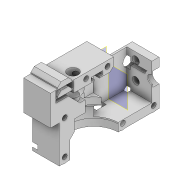
# Autodesk Inventor part: 10_SOOCT_Base_v3
Saved by Autodesk Inventor 2022 (Build 260153000, 153)
## iProperties
Created: 2023-01-02
Part Number: 10_SOOCT_Base_v3
Material: Generisch
Document SubType Name: Modeling
Designer: diederichbenedict
Density: 1 g/cm^3
Appearance: Vorgabe
Author: diederichbenedict
Autodesk Inventor part; units mm, degrees
ref_plane "YZ Plane" through (0, 0, 0) normal (1, 0, 0) x (0, 1, 0)
ref_plane "XZ Plane" through (0, 0, 0) normal (0, 1, 0) x (-1, 0, 0)
ref_plane "XY Plane" through (0, 0, 0) normal (0, 0, 1) x (1, 0, 0)
ref_plane "Arbeitsebene1" through (-39.7131, -1.3218, -40.6417) normal (-1, 0, 0) x (0, 0, -1)
sketch "Skizze1" plane through (-39.7131, -1.3218, -40.6417) normal (-1, 0, 0) x (0, 0, -1)
  line L0 (-10.1, 42.0592) -> (-10.1, 20.2092)
  line L1 (-10.1, 19.2092) -> (-10.1, 18.0592)
  line L2 (-37.1, 42.0592) -> (-37.1, 20.2092)
  line L3 (-37.1, 19.2092) -> (-37.1, 18.0592)
  line L4 (4, 5) -> (1, 5)
  line L5 (-37.1, 27.2) -> (-43.1, 27.2)
  line L6 (-43.1, 27.2) -> (-43.1, 3.2)
  line L7 (-43.1, 3.2) -> (-37.1, 3.2)
  line L8 (-37.1, 3.2) -> (-37.1, 27.2)
  line L9 (-7.8, 3.2) -> (0, 3.2)
  line L10 (-37.1, 3.2) -> (12.9, 3.2)
  line L11 (12.9, 3.2) -> (12.9, 27.2)
  line L12 (12.9, 27.2) -> (-37.1, 27.2)
  line L13 (-37.1, 27.2) -> (-37.1, 3.2)
  point P0 (-40.6417, -1.3218)
  point P1 (-37.1, 24.2092)
  point P2 (-7.8, 3.2)
  dimension "d0" = 0
  dimension "d2" = 6
  dimension "d3" = 50
  dimension "d21" = 24
  constraints: 28 end point, 4 horizontal, 4 parallel, 4 vertical, 2 perpendicular, 1 point on line, 12 other
  measures "d0" distance between parallel lines of L7 L9
  measures "d2" distance between parallel lines of L8 L6
  measures "d3" distance of L5.start L11.end
  measures "d21" distance between parallel lines of L12 L7
extrude "Extrusion1" add sketch "Skizze1" against normal up to surface (17 mm away)
sketch "Skizze2" plane through (-22.7131, -28.5218, 2.4583) normal (1, 0, 0) x (0, 0, -1)
  line L0 (33, 5) -> (33, 6.15)
  line L1 (33, -17.85) -> (33, 4)
  line L2 (0, 24) -> (56, 24)
  line L3 (8.5007, 24) -> (8.5007, 11.4732)
  line L4 (8.5007, 11.4732) -> (5.9, 8.8725)
  line L5 (5.9, 8.8725) -> (5.9, 7.6275)
  arc A0 (5.9, 6.8275) -> (5.9, 7.6275) centre (5.9, 7.2275) ccw
  line L6 (5.9, 6.8275) -> (5.9, -14.594)
  line L7 (56.2565, 0) -> (0.3327, 0)
  line L8 (15.7023, 20.4) -> (24.9625, 20.4029)
  line L9 (19.4614, 24) -> (19.4689, 0)
  line L10 (33, 7.9908) -> (6, 7.9908) projected
  line L11 (33, 6.9908) -> (6, 6.9908) projected
  line L12 (56, 24) -> (0, 24) projected
  line L13 (6, 7.9908) -> (6, 9.1408)
  line L14 (56, 0) -> (56, 24) projected
  line L15 (56, 24) -> (0, 24) projected
  line L16 (0, 24) -> (0, 0) projected
  line L17 (0, 0) -> (56, 0) projected
  line L18 (5.9662, 8.7775) -> (13.9636, 16.7801)
  line L19 (5.9, 7.6275) -> (5.9, 6.8275)
  point P0 (2.4583, 28.5218)
  point P1 (5.9, 0)
  point P2 (7.3142, 24)
  dimension "d10" = 5.5
  dimension "d37" = 0
  dimension "d38" = 0.1
  dimension "d39" = 0
  dimension "d40" = 0.8
  constraints: 26 end point, 6 point on line, 2 collinear, 2 point on circle, 1 centre point, 1 coincident, 1 parallel, 1 vertical, 4 other
  measures "d10" distance from line of L8.end L9
  measures "d37" distance between parallel lines of L12 L2
  measures "d38" distance between parallel lines of L13 L5
  measures "d39" distance between parallel lines of L6 L5
  measures "d40" distance of L5.end L6.start
revolve "Umdrehung1" cut sketch "Skizze2" angle 360 about axis through (-22.7131, -4.5218, -17.0031) along (0, -1, -0.0003154) contours L2 L9 L10 L13 L4 L3 | L13 L10 L9 L11 A0 L5 L4 | L6 A0 L11 L9 L7 | L19 A0
sketch "Skizze3" plane through (-22.7131, -28.5218, -53.5417) normal (1, 0, 0) x (0, 0, -1)
  line L0 (-38.5, 18.2) -> (-38.5, 22.2) projected
  line L1 (-34.5, 18.2) -> (-38.5, 18.2) projected
  line L2 (-34.5, 22.2) -> (-34.5, 18.2) projected
  line L3 (-38.5, 22.2) -> (-34.5, 22.2) projected
  line L4 (-34, 22.7) -> (-34, 17.7)
  line L5 (-34, 17.7) -> (-39, 17.7)
  line L6 (-39, 17.7) -> (-39, 22.7)
  line L7 (-39, 22.7) -> (-34, 22.7)
  line L8 (-47.4993, 11.4732) -> (-47.4993, 24) projected
  line L9 (-25.578, 24) -> (-25.5701, 11.4801) projected
  line L10 (-47.4993, 22.7) -> (-25.574, 22.7)
  line L11 (-25.574, 22.7) -> (-25.574, 17.7)
  line L12 (-25.574, 17.7) -> (-47.4993, 17.7)
  line L13 (-47.4993, 17.7) -> (-47.4993, 22.7)
  line L14 (-47.4993, 22.7) -> (-25.578, 22.7)
  line L15 (-25.578, 22.7) -> (-25.578, 24)
  line L16 (-25.578, 24) -> (-47.4993, 24)
  line L17 (-47.4993, 24) -> (-47.4993, 22.7)
  point P0 (-53.5417, 28.5218)
  point P1 (-47.4993, 17.7)
  point P2 (-34, 14.7092)
  point P3 (-25.5771, 22.7)
  point P4 (-34, 19.7092)
  point P5 (-34, 19.7092)
  point P6 (-34, 22.7)
  point P7 (-34, 17.7)
  point P8 (-47.4993, 24)
  point P9 (-25.578, 22.7)
  dimension "d12" = 0.5
  constraints: 24 end point, 4 parallel, 4 point on line, 2 horizontal, 2 perpendicular, 3 other
  measures "d12" distance between parallel lines of L3 L7
extrude "Extrusion2" add sketch "Skizze3" against normal through all contours L0 L3 L2 L1 | L10 L9 L12 L4 | L4 L5 L6 L7 | L7 L10 L8 L16 L9 | L6 L12 L8 L10 | L10 L11 L9
sketch "Skizze4" plane through (-22.7131, -28.5218, -53.5417) normal (1, 0, 0) x (0, 0, -1)
  line L0 (-38.5, 18.2) -> (-38.5, 22.2) projected
  line L1 (-34.5, 18.2) -> (-38.5, 18.2) projected
  line L2 (-34.5, 22.2) -> (-34.5, 18.2) projected
  line L3 (-38.5, 22.2) -> (-34.5, 22.2) projected
  line L4 (-34.45, 22.25) -> (-34.45, 18.15)
  line L5 (-34.45, 18.15) -> (-38.55, 18.15)
  line L6 (-38.55, 18.15) -> (-38.55, 22.25)
  line L7 (-38.55, 22.25) -> (-34.45, 22.25)
  line L8 (-56, 0) -> (-50.1, 0) projected
  line L9 (0, 0) -> (0, 24) projected
  line L10 (0, 24) -> (-25.578, 24) projected
  line L11 (-56, 24) -> (-56, 0) projected
  line L12 (-38.2, 22.25) -> (-34.8, 22.25)
  line L13 (-34.8, 22.25) -> (-34.8, 22.7)
  line L14 (-34.8, 22.7) -> (-38.2, 22.7)
  line L15 (-38.2, 22.7) -> (-38.2, 22.25)
  line L16 (-34.5, 18.2) -> (-34.5, 22.2)
  line L17 (-38.25, 18.15) -> (-34.75, 18.15)
  line L18 (-34.75, 18.15) -> (-34.75, 17.7)
  line L19 (-34.75, 17.7) -> (-38.25, 17.7)
  line L20 (-38.25, 17.7) -> (-38.25, 18.15)
  line L21 (-25.578, 24) -> (-25.5771, 22.7) projected
  line L22 (-25.5701, 11.4801) -> (-22.9677, 8.8811) projected
  line L23 (-47.4993, 11.4732) -> (-47.4993, 17.7) projected
  line L24 (-50.1, 8.8725) -> (-47.4993, 11.4732) projected
  line L25 (-47.4993, 17.7) -> (-25.574, 17.7) projected
  line L26 (-25.574, 17.7) -> (-25.5701, 11.4801) projected
  line L27 (-25.5771, 22.7) -> (-25.578, 22.7) projected
  line L28 (-22.9621, 0.0086) -> (-36.5311, 0) projected
  line L29 (-36.5311, 0) -> (0, 0) projected
  line L30 (-25.578, 22.7) -> (-25.578, 24) projected
  line L31 (-25.578, 24) -> (-56, 24) projected
  line L32 (-38.2, 22.7) -> (-34.8, 22.7)
  line L33 (-34.8, 22.7) -> (-34.8, 24)
  line L34 (-34.8, 24) -> (-38.2, 24)
  line L35 (-38.2, 24) -> (-38.2, 22.7)
  line L36 (-34.45, 21.95) -> (-21.9312, 21.95)
  line L37 (-21.9312, 21.95) -> (-21.9312, 18.5)
  line L38 (-21.9312, 18.5) -> (-34.45, 18.5)
  line L39 (-34.45, 18.5) -> (-34.45, 21.95)
  line L40 (-50.1, 0) -> (-50.1, 8.8725) projected
  line L41 (-22.9677, 8.8811) -> (-22.9621, 0.0086) projected
  point P0 (-53.5417, 28.5218)
  point P1 (-43.6858, 14.7092)
  point P2 (-19.3142, 14.7092)
  point P3 (-47.4993, 22.7)
  point P4 (-34.75, 18.15)
  point P5 (-34.8059, 22.7)
  point P6 (-34.45, 18.5)
  dimension "d15" = 0.05
  dimension "d58" = 0.3
  dimension "d59" = 0.3
  dimension "d60" = 0.3
  dimension "d61" = 0.3
  dimension "d64" = 0.3
  dimension "d65" = 0.3
  constraints: 42 end point, 8 parallel, 5 point on line, 4 horizontal, 4 perpendicular, 3 other
  measures "d15" distance between parallel lines of L3 L7
  measures "d58" distance between parallel lines of L0 L15
  measures "d59" distance between parallel lines of L2 L33
  measures "d60" distance between parallel lines of L4 L18
  measures "d61" distance between parallel lines of L20 L6
  measures "d64" distance between parallel lines of L7 L36
  measures "d65" distance between parallel lines of L38 L1
extrude "Extrusion3" cut sketch "Skizze4" against normal blind 2 contours L0 L3 L2 L1 | L4 L5 L6 L7 | L36 L37 L38 L4 | L7 L15 L14 L13 | L14 L35 L31 L33 | L18 L19 L20 L5
sketch "Skizze5" plane through (-39.7131, -28.5218, -53.5417) normal (0, 0, -1) x (-1, 0, 0)
  arc A0 (-8, 26.2) -> (-9, 27.2) centre (-9, 26.2) ccw projected
  line L0 (-25, 27.2) -> (-9, 27.2) projected
  arc A1 (-25, 27.2) -> (-26, 26.2) centre (-25, 26.2) ccw projected
  line L1 (-26, 10.2) -> (-26, 26.2) projected
  arc A2 (-26, 10.2) -> (-25, 9.2) centre (-25, 10.2) ccw projected
  line L2 (-9, 9.2) -> (-25, 9.2) projected
  arc A3 (-9, 9.2) -> (-8, 10.2) centre (-9, 10.2) ccw projected
  line L3 (-8, 26.2) -> (-8, 10.2) projected
  circle A4 centre (-17, 18.2) radius 5.8 projected
  arc A5 (-9, 8.2) -> (-7, 10.2) centre (-9, 10.2) ccw
  line L4 (-9, 8.2) -> (-25, 8.2)
  arc A6 (-27, 10.2) -> (-25, 8.2) centre (-25, 10.2) ccw
  line L5 (-27, 10.2) -> (-27, 26.2)
  arc A7 (-25, 28.2) -> (-27, 26.2) centre (-25, 26.2) ccw
  line L6 (-25, 28.2) -> (-9, 28.2)
  arc A8 (-7, 26.2) -> (-9, 28.2) centre (-9, 26.2) ccw
  line L7 (-7, 26.2) -> (-7, 10.2)
  line L8 (-31, 32.2) -> (-3, 32.2)
  line L9 (-3, 32.2) -> (-3, 4.2)
  line L10 (-3, 4.2) -> (-31, 4.2)
  line L11 (-31, 4.2) -> (-31, 32.2)
  line L12 (-31, 32.2) -> (-3, 4.2) construction
  line L13 (-3, 32.2) -> (-31, 4.2) construction
  point P0 (-39.7131, 28.5218)
  dimension "d18" = 1
  dimension "d27" = 28
  dimension "d28" = 28
  constraints: 20 end point, 8 point on circle, 4 centre point, 2 midpoint, 2 parallel, 1 horizontal, 1 perpendicular, 7 other
  measures "d18" distance between parallel lines of L3 L7
  measures "d27" distance of L9.end L10.end
  measures "d28" distance of L8.end L9.end
extrude "Extrusion4" cut sketch "Skizze5" against normal blind 20 contours L3 A3 L2 A2 L1 A1 L0 A0 | A4 | L4 A6 L5 A7 L6 A8 L7 A5
sketch "Skizze6" plane through (-39.7131, -28.5218, -53.5417) normal (0, 0, -1) x (-1, 0, 0)
  line L0 (-9, 8.2) -> (-17, 8.2) projected
  line L1 (-17, 0) -> (-17, 8.2) projected
  line L2 (0, 0) -> (-17, 0) projected
  line L3 (0, 24) -> (0, 0) projected
  line L4 (0, 24) -> (-7, 24) projected
  line L5 (-7, 24) -> (-7, 10.2) projected
  arc A0 (-9, 8.2) -> (-7, 10.2) centre (-9, 10.2) ccw projected
  line L6 (-17, 8.2) -> (-17, 11.4801) projected
  line L7 (-17, 8.2) -> (-7, 8.2)
  line L8 (-7, 8.2) -> (-7, 24)
  line L9 (-7, 24) -> (-17, 24)
  line L10 (-17, 24) -> (-17, 8.2)
  circle A1 centre (-17, 18.2) radius 4 projected
  circle A2 centre (-17, 15.0113) radius 4
  point P0 (-39.7131, 28.5218)
  point P1 (-17, 22.2)
  point P2 (-17, 14.2)
  point P3 (-17, 19.0113)
  point P4 (-17, 11.0113)
  constraints: 8 end point, 2 parallel, 1 centre point, 1 horizontal, 1 perpendicular, 2 other
ref_plane "Arbeitsebene2" through (-26.7131, -14.3218, -41.6417) normal (0, 0, 1) x (1, 0, 0)
ref_plane "Arbeitsebene3" through (-26.7131, -14.3218, -44.6417) normal (0, 0, -1) x (0, 1, 0)
extrude "Extrusion5" add sketch "Skizze6" against normal blind 8 contours L0 L6 A2 A1 L10 L9 L5 A0 | A1 A2 L10 picked at (-16.3965, 20.005)
sketch "Skizze7" plane through (-32.7131, -4.5218, -45.5417) normal (0, 0, 1) x (1, 0, 0)
  circle A0 centre (10, -5.8) radius 4
  line L0 (10, 0) -> (10, -24) projected
  line L1 (10, -9.8) -> (10, -1.8)
  circle A1 centre (10, -5.8) radius 3
  circle A2 centre (10, -8.9887) radius 4 projected
  point P0 (32.7131, 4.5218)
  point P1 (10, -8.8)
  point P2 (10, -2.8)
  dimension "d24" = 1
  constraints: 2 centre point, 2 end point, 1 point on circle
  measures "d24" radial gap between concentric circles of A0 A1
extrude "Extrusion6" add sketch "Skizze7" against normal blind 0.5 contours L0 A1 A2 A0 | A2 A1 L0 A0 picked at (9.6732, -2.174) picked at (9.6932, -9.4309)
ref_plane "Arbeitsebene4" through (-39.7131, -28.5218, -35.5417) normal (0, 0, -1) x (-1, 0, 0)
sketch "Skizze8" plane through (-39.7131, -28.5218, -35.5417) normal (0, 0, -1) x (-1, 0, 0)
  circle A0 centre (-17, 18.2) radius 4 projected
  line L0 (-3, 3.7) -> (-31, 3.7)
  line L1 (-31, 3.7) -> (-31, 32.7)
  line L2 (-31, 32.7) -> (-3, 32.7)
  line L3 (-3, 32.7) -> (-3, 3.7)
  line L4 (-17, 22.2) -> (-17, 18.2) projected
  line L5 (-3, 3.7) -> (-31, 32.7) construction
  line L6 (-31, 3.7) -> (-3, 32.7) construction
  point P0 (-39.7131, 28.5218)
  dimension "d30" = 28
  dimension "d31" = 29
  constraints: 12 end point, 2 midpoint, 2 parallel, 1 horizontal, 1 perpendicular, 1 vertical alignment
  measures "d30" distance of L1.end L2.end
  measures "d31" distance of L0.end L1.end
extrude "Extrusion7" cut sketch "Skizze8" along normal blind 14 and the other way blind 9 contours A0 | L0 L1 L2 L3
sketch "Skizze9" plane through (-39.7131, -28.5218, -53.5417) normal (0, 0, -1) x (-1, 0, 0)
  line L0 (-17, 11.0113) -> (-17, 0) projected
  line L1 (0, 0) -> (-17, 0) projected
  line L2 (0, 24) -> (0, 0) projected
  line L3 (0, 24) -> (-17, 24) projected
  line L4 (-17, 24) -> (-17, 19.0113) projected
  arc A0 (-17, 11.0113) -> (-17, 19.0113) centre (-17, 15.0113) ccw projected
  line L5 (-26, 10.0113) -> (-8, 10.0113)
  line L6 (-8, 10.0113) -> (-8, 20.0113)
  line L7 (-8, 20.0113) -> (-26, 20.0113)
  line L8 (-26, 20.0113) -> (-26, 10.0113)
  line L9 (-26, 10.0113) -> (-8, 20.0113) construction
  line L10 (-8, 10.0113) -> (-26, 20.0113) construction
  circle A1 centre (-8, 20.0113) radius 2
  circle A2 centre (-8, 10.0113) radius 2
  point P0 (-39.7131, 28.5218)
  dimension "d99" = 18
  dimension "d100" = 10
  dimension "d101" = 4
  dimension "d102" = 4
  constraints: 12 end point, 2 centre point, 2 coincident, 2 midpoint, 2 parallel, 1 horizontal, 1 perpendicular
  measures "d99" distance of L7.end L6.end
  measures "d100" distance of L6.end L5.end
  measures "d101" diameter of A1
  measures "d102" diameter of A2
extrude "Extrusion8" cut sketch "Skizze9" against normal blind 14 contours A2 L6 L5 | L5 L6 A2 | A1 L6 L7 | L7 L6 A1
sketch "Skizze10" plane through (-39.7131, -28.5218, -53.5417) normal (0, -1, 0) x (1, 0, 0)
  line L0 (8.5019, 6.0924) -> (3.4981, 6.0924) projected
  line L1 (17, 56) -> (17, 50.1) projected
  line L2 (0, 56) -> (17, 56) projected
  line L3 (0, 0) -> (0, 56) projected
  line L4 (0, 0) -> (17, 0) projected
  line L5 (17, 36.5311) -> (17, 0) projected
  line L6 (17, 50.1) -> (17, 36.5311) projected
  ellipse E0 centre (17, 36.5311) end of major axis (30.5689, 36.5311) minor radius 13.5689 (17, 50.1) -> (17, 22.9621) ccw projected
  point P0 (39.7131, 53.5417)
  constraints: 1 other
extrude "Extrusion9" cut sketch "Skizze10" against normal blind 3 contours L6 L5 E0
sketch "Skizze11" plane through (-39.7131, -28.5218, -53.5417) normal (0, -1, 0) x (1, 0, 0)
  circle A0 centre (17, 36.5) radius 13.5 projected
  ellipse E0 centre (17, 36.5311) end of major axis (30.5689, 36.5311) minor radius 13.5689 (17, 50.1) -> (17, 22.9621) ccw projected
  line L0 (17, 56) -> (17, 50.1) projected
  line L1 (0, 56) -> (17, 56) projected
  line L2 (0, 0) -> (0, 56) projected
  line L3 (0, 0) -> (17, 0) projected
  line L4 (17, 22.9621) -> (17, 0) projected
  point P0 (39.7131, 53.5417)
  constraints: 1 other
extrude "Extrusion10" add sketch "Skizze11" along normal blind 3 contours E0 L4 L3 L2 L1 L0
sketch "Skizze12" plane through (-39.7131, -1.3218, -40.6417) normal (-1, 0, 0) x (0, 0, 1)
  circle A0 centre (40.1, -25.2) radius 1.29
  circle A1 centre (40.1, -6.2) radius 1.4
  circle A2 centre (-9.9, -25.2) radius 1.4
  circle A3 centre (7.4249, -25.2) radius 1.4
  circle A4 centre (-9.9, -10.2) radius 1.4
  line L0 (43.1, -30.2) -> (-12.9, -30.2) projected
  line L1 (43.1, -30.2) -> (43.1, -3.2) projected
  line L2 (-12.9, -3.2) -> (-12.9, -30.2) projected
  line L3 (43.1, -3.2) -> (-12.9, -3.2) projected
  point P0 (40.6417, 1.3218)
  dimension "d46" = 2.58
  dimension "d47" = 2.8
  dimension "d48" = 2.8
  dimension "d49" = 2.8
  dimension "d50" = 2.8
  dimension "d90" = 3
  dimension "d91" = 3
  dimension "d92" = 3
  dimension "d93" = 5
  dimension "d94" = 5
  dimension "d95" = 5
  dimension "d96" = 3
  dimension "d97" = 7
  dimension "d98" = 3
  constraints: 5 centre point
  measures "d46" diameter of A0
  measures "d47" diameter of A1
  measures "d48" diameter of A2
  measures "d49" diameter of A3
  measures "d50" diameter of A4
  measures "d90" distance from line of A0.centre L1
  measures "d91" distance from line of A1.centre L1
  measures "d92" distance from line of L3 A1.centre
  measures "d93" distance from line of L0 A0.centre
  measures "d94" distance from line of L0 A3.centre
  measures "d95" distance from line of L0 A2.centre
  measures "d96" distance from line of A4.centre L2
  measures "d97" distance from line of A4.centre L3
  measures "d98" distance from line of L2 A2.centre
hole "Bohrung1" at (-39.7131, -26.5218, -0.5417) at (-39.7131, -7.5218, -0.5417) at (-39.7131, -26.5218, -33.2168) at (-39.7131, -26.5218, -50.5417) at (-39.7131, -11.5218, -50.5417) direction (1, 0, 0) diameter 2.8 end through all counterbore diameter 6.5 counterbore depth 5
sketch "Skizze13" plane through (-39.7131, -1.3218, -40.6417) normal (-1, 0, 0) x (0, 0, 1)
  line L0 (37.2, -30.2) -> (43.1, -30.2) projected
  line L1 (43.1, -30.2) -> (-14.489, -30.2)
  line L2 (-14.489, -30.2) -> (-14.489, -1.9274)
  line L3 (-14.489, -1.9274) -> (43.1, -1.9274)
  line L4 (43.1, -1.9274) -> (43.1, -30.2)
  point P0 (40.6417, 1.3218)
  point P1 (37.2, -30.2)
  constraints: 8 end point, 2 parallel, 1 horizontal, 1 perpendicular
extrude "Extrusion11" cut sketch "Skizze13" against normal blind 2
sketch "Skizze14" plane through (-39.7131, -28.5218, -49.5417) normal (0, 0, 1) x (1, 0, 0)
  arc A0 (17, 19.0113) -> (17, 11.0113) centre (17, 15.0113) ccw projected
  circle A1 centre (17, 15.0113) radius 2.5
  line L0 (17, 11.0113) -> (17, 3.7) projected
  line L1 (17, 11.0113) -> (17, 19.0113)
  point P0 (39.7131, 28.5218)
  point P1 (17, 9.4504)
  point P2 (17, 12.5113)
  point P3 (17, 17.5113)
  dimension "d68" = 5
  constraints: 2 end point, 1 centre point, 1 coincident, 1 collinear
  measures "d68" diameter of A1
extrude "Extrusion12" add sketch "Skizze14" against normal blind 0.5 contours L1 A1 A0
sketch "Skizze15" plane through (-37.7131, -1.3218, -40.6417) normal (-1, 0, 0) x (0, 0, 1)
  circle A0 centre (7.4249, -25.2) radius 3.25 projected
  arc A1 (38.85, -3.2) -> (43.1, -7.45) centre (40.1, -6.2) ccw projected
  line L0 (43.1, -3.2) -> (43.1, -4.95) projected
  line L1 (-12.9, -8.95) -> (-12.9, -3.2) projected
  line L2 (-12.9, -30.2) -> (-12.9, -26.45) projected
  line L3 (43.1, -26.45) -> (43.1, -30.2) projected
  line L4 (43.1, -3.2) -> (43.1, -30.2) projected
  line L5 (-12.9, -30.2) -> (43.1, -30.2)
  line L6 (43.1, -30.2) -> (43.1, -28.2)
  line L7 (43.1, -28.2) -> (-12.9, -28.2)
  line L8 (-12.9, -28.2) -> (-12.9, -30.2)
  arc A2 (43.1, -4.95) -> (41.35, -3.2) centre (40.1, -6.2) ccw projected
  arc A3 (-12.9, -11.45) -> (-12.9, -8.95) centre (-9.9, -10.2) ccw projected
  line L9 (41.35, -3.2) -> (43.1, -3.2) projected
  arc A4 (43.1, -23.95) -> (43.1, -26.45) centre (40.1, -25.2) ccw projected
  line L10 (43.1, -30.2) -> (-12.9, -30.2) projected
  line L11 (43.1, -7.45) -> (43.1, -23.95) projected
  line L12 (-12.9, -3.2) -> (38.85, -3.2) projected
  arc A5 (-12.9, -26.45) -> (-12.9, -23.95) centre (-9.9, -25.2) ccw projected
  line L13 (-12.9, -23.95) -> (-12.9, -11.45) projected
  point P0 (40.6417, 1.3218)
  point P1 (6.1749, -28.2)
  point P2 (8.6749, -28.2)
  point P3 (41.35, -30.2)
  point P4 (43.1, -28.45)
  point P5 (0.4177, -30.2)
  point P6 (2.9177, -30.2)
  point P7 (2.9177, -30.2)
  point P8 (-12.9, -28.45)
  point P9 (-11.15, -30.2)
  point P10 (-8.65, -28.2)
  point P11 (-11.15, -28.2)
  point P12 (41.35, -28.2)
  point P13 (38.85, -28.2)
  dimension "d71" = 2
  constraints: 8 end point, 2 parallel, 1 horizontal, 1 perpendicular, 1 point on line
  measures "d71" distance of L6.end L5.end
extrude "Extrusion13" cut sketch "Skizze15" against normal through all contours A0 L7 A4 L3 L5 L2 A5
sketch "Skizze16" plane through (-22.7131, -20.8943, -3.4417) normal (1, 0, 0) x (0, 0, -1)
  circle A0 centre (13.6, 12.5725) radius 4.6
  line L0 (50.1, 16.3725) -> (-5.9, 16.3725) projected
  line L1 (9.9503, 16.3725) -> (9.9503, 15.3725)
  line L2 (9.9503, 16.3725) -> (10.9503, 16.3725) construction
  line L3 (17.2497, 16.3725) -> (17.2497, 15.3725)
  line L4 (11.55, 14.6225) -> (15.65, 10.5225)
  line L5 (15.65, 10.5225) -> (15.65, 14.6225)
  line L6 (15.65, 14.6225) -> (11.55, 10.5225)
  point P0 (-3.4417, 20.8943)
  point P1 (16.1923, 16.3725)
  point P2 (11.0077, 16.3725)
  dimension "d74" = 9.2
  dimension "d80" = 90
  dimension "d81" = 1
  dimension "d82" = 1
  constraints: 12 end point, 3 midpoint, 2 perpendicular, 2 point on circle, 2 point on line, 2 vertical, 1 centre point, 1 horizontal
  measures "d74" diameter of A0
  measures "d80" angle of L1 L2
  measures "d81" distance of L1.end L1.start
  measures "d82" distance from line of L3.end L0
extrude "Extrusion14" cut sketch "Skizze16" against normal blind 13 contours A0 L0 | A0 L0 L3 | L1 L0 A0 | L0 A0 | L6 L5 L4
ref_plane "Arbeitsebene5" through (-32.7131, -12.3218, -21.0417) normal (1, 0, 0) x (0, 1, 0)
sketch "Skizze18" plane through (-22.7131, -20.8943, -3.4417) normal (1, 0, 0) x (0, 0, -1)
  line L0 (9.9503, 15.3725) -> (9.9503, 16.3725) projected
  line L1 (9.9503, 16.3725) -> (-5.9, 16.3725) projected
  line L2 (-5.9, 16.3725) -> (-5.9, -8.6275) projected
  line L3 (0, -4.6275) -> (0, -8.6275) projected
  line L4 (0, 1.245) -> (2.6007, 3.8457) projected
  line L5 (2.6007, 3.8457) -> (2.6007, 10.0725) projected
  line L6 (2.6007, 10.0725) -> (9.7387, 10.0725) projected
  arc A0 (9.9503, 15.3725) -> (9.7387, 10.0725) centre (13.6, 12.5725) ccw projected
  circle A1 centre (-2.9, -5.6275) radius 1.4 projected
  circle A2 centre (-2.9, 13.3725) radius 1.4 projected
  line L7 (18.5632, 7.5725) -> (8.5632, 7.5725)
  line L8 (8.5632, 7.5725) -> (8.5632, 17.5725)
  line L9 (8.5632, 17.5725) -> (18.5632, 17.5725)
  line L10 (18.5632, 17.5725) -> (18.5632, 7.5725)
  line L11 (18.5632, 7.5725) -> (8.5632, 17.5725) construction
  line L12 (8.5632, 7.5725) -> (18.5632, 17.5725) construction
  line L13 (50.1, 3.3838) -> (50.1, -8.6275) projected
  line L14 (46.1, -3.9275) -> (46.1, 4.8838) projected
  line L15 (46.1, -3.9275) -> (27.1355, -3.9275) projected
  line L16 (27.1355, -3.9275) -> (27.136, -4.6275) projected
  line L17 (27.136, -4.6275) -> (27.1379, -4.6275) projected
  line L18 (27.1379, -4.6275) -> (27.1379, -8.6275) projected
  circle A3 centre (29.7751, -5.6275) radius 1.4 projected
  circle A4 centre (47.1, -5.6275) radius 1.4 projected
  line L19 (50.1, 3.3838) -> (46.6, 3.3838) projected
  line L20 (46.6, 4.8838) -> (46.6, 3.3838) projected
  line L21 (46.1, 4.8838) -> (46.6, 4.8838) projected
  line L22 (48.35, -8.6275) -> (50.1, -8.6275) projected
  line L23 (27.1379, -8.6275) -> (28.5251, -8.6275) projected
  arc A5 (28.5251, -8.6275) -> (31.0251, -8.6275) centre (29.7751, -5.6275) ccw projected
  line L24 (31.0251, -8.6275) -> (45.85, -8.6275) projected
  arc A6 (45.85, -8.6275) -> (48.35, -8.6275) centre (47.1, -5.6275) ccw projected
  line L25 (-5.9, -8.6275) -> (-4.15, -8.6275) projected
  arc A7 (-4.15, -8.6275) -> (-1.65, -8.6275) centre (-2.9, -5.6275) ccw projected
  line L26 (-1.65, -8.6275) -> (0, -8.6275) projected
  line L27 (18.5632, 7.5725) -> (24.0476, 7.5725)
  line L28 (24.0476, 7.5725) -> (24.0476, 17.5725)
  line L29 (24.0476, 17.5725) -> (18.5632, 17.5725)
  line L30 (18.5632, 17.5725) -> (18.5632, 7.5725)
  line L31 (0, -4.6275) -> (0, 1.245) projected
  point P0 (-3.4417, 20.8943)
  point P1 (13.5632, 12.5725)
  point P2 (8.5632, 10.0725)
  point P3 (8.5632, 16.3725)
  dimension "d83" = 10
  dimension "d84" = 10
  constraints: 20 end point, 4 parallel, 2 horizontal, 2 midpoint, 2 perpendicular
  measures "d83" distance of L8.end L9.end
  measures "d84" distance of L7.end L8.end
extrude "Extrusion16" cut sketch "Skizze18" against normal up to surface (10 mm away) contours A0 L6 L8 L1 L0 | L0 L1 L8 L9 L10 L7 L6 A0 | L29 L28 L27 L10
sketch "Skizze19" plane through (-37.7131, -1.3218, -40.6417) normal (-1, 0, 0) x (0, 0, 1)
  circle A0 centre (23.6, -7) radius 1.5 projected
  circle A1 centre (23.6, -7) radius 1.6
  point P0 (40.6417, 1.3218)
  dimension "d87" = 3.2
  constraints: 1 centre point, 1 coincident
  measures "d87" diameter of A1
extrude "Extrusion17" cut sketch "Skizze19" against normal through all contours A0 | A1
sketch "Skizze20" plane through (-34.7131, -8.7718, 2.4583) normal (0, 0, 1) x (1, 0, 0)
  line L0 (2.55, -2.9214) -> (5.65, -2.9214) construction
  line L1 (5.65, -2.9214) -> (2.55, -2.9214) projected
  line L2 (2.2436, -4.55) -> (2.2441, -2.05) projected
  line L3 (2.2441, -2.05) -> (12, -2.05) projected
  line L4 (2.55, -2.9214) -> (2.55, 0.1786) construction
  line L5 (2.55, 0.1786) -> (5.65, 0.1786) projected
  line L6 (12, 4.25) -> (12, -20.75) projected
  line L7 (-3, 4.25) -> (12, 4.25) projected
  line L8 (-3, 4.25) -> (-3, 2.5) projected
  line L9 (-3, 2.5) -> (0, 2.5) projected
  line L10 (0, 2.5) -> (0, 0) projected
  line L11 (0, 0) -> (-3, 0) projected
  line L12 (-3, 0) -> (-3, -16.5) projected
  line L13 (-3, -16.5) -> (0, -16.5) projected
  line L14 (0, -16.5) -> (0, -19) projected
  line L15 (5.65, 0.1786) -> (5.65, -2.9214) projected
  circle A0 centre (4.1, -1.7586) radius 1.55
  circle A1 centre (4.1, -1.7586) radius 2
  line L16 (14.05, -1.65) -> (9.95, -1.65) projected
  line L17 (9.95, 2.55) -> (9.95, -1.65) projected
  line L18 (9.95, 2.55) -> (14.05, 2.55) projected
  line L19 (14.05, 2.55) -> (14.05, -1.65) projected
  line L20 (0, -19) -> (-3, -19) projected
  line L21 (-3, -19) -> (-3, -20.75) projected
  line L22 (-3, -20.75) -> (12, -20.75) projected
  point P0 (34.7131, 8.7718)
  point P1 (5.8244, -2.15)
  point P2 (2.8244, -2.15)
  dimension "d103" = 4
  constraints: 2 centre point, 2 end point, 1 coincident, 6 other
  measures "d103" diameter of A1
extrude "Extrusion18" cut sketch "Skizze20" against normal up to surface (14.4632 mm away) contours L15 L3 A1 L2 A0 L1 | L1 A0 L3 L15 | A0 L1 | L1 A0 L3 | L15 A1 L3 | L3 A0 L15 | L3 A0 | A0 L3 L2 A1 L5 L15 | A1 L5
sketch "Skizze21" plane through (-37.7131, -1.3218, -40.6417) normal (-1, 0, 0) x (0, 0, 1)
  circle A0 centre (23.6, -7) radius 1.6 projected
  line L0 (-8.65, -28.2) -> (6.1749, -28.2) projected
  arc A1 (8.6749, -28.2) -> (6.1749, -28.2) centre (7.4249, -25.2) ccw projected
  line L1 (8.6749, -28.2) -> (38.85, -28.2) projected
  arc A2 (43.1, -23.95) -> (38.85, -28.2) centre (40.1, -25.2) ccw projected
  line L2 (43.1, -7.45) -> (43.1, -23.95) projected
  arc A3 (38.85, -3.2) -> (43.1, -7.45) centre (40.1, -6.2) ccw projected
  line L3 (-12.9, -3.2) -> (38.85, -3.2) projected
  line L4 (-12.9, -8.95) -> (-12.9, -3.2) projected
  arc A4 (-12.9, -11.45) -> (-12.9, -8.95) centre (-9.9, -10.2) ccw projected
  line L5 (-12.9, -23.95) -> (-12.9, -11.45) projected
  arc A5 (-8.65, -28.2) -> (-12.9, -23.95) centre (-9.9, -25.2) ccw projected
  line L6 (36.1, 6.1) -> (38.1, 8.1)
  line L7 (36.1, 5.5) -> (36.1, 6.1)
  line L8 (35.1, 5.5) -> (36.1, 5.5)
  line L9 (35.1, 9.3) -> (35.1, 5.5)
  line L10 (45.1, 9.3) -> (35.1, 9.3)
  line L11 (45.1, 5.5) -> (45.1, 9.3)
  line L12 (44.1, 5.5) -> (45.1, 5.5)
  line L13 (44.1, 6.1) -> (44.1, 5.5)
  line L14 (42.1, 8.1) -> (44.1, 6.1)
  line L15 (38.1, 8.1) -> (42.1, 8.1)
  line L16 (42.1, 12.3) -> (44.1, 10.3)
  line L17 (38.1, 12.3) -> (42.1, 12.3)
  line L18 (36.1, 10.3) -> (38.1, 12.3)
  line L19 (36.1, 9.7) -> (36.1, 10.3)
  line L20 (36.1, 9.7) -> (12.6, 9.7)
  line L21 (12.6, 5.2) -> (12.6, 9.7)
  line L22 (35.1, 3.3) -> (29.5691, 3.3)
  line L23 (35.1, 5.1) -> (35.1, 3.3)
  line L24 (45.1, 5.1) -> (35.1, 5.1)
  line L25 (45.1, 3.3) -> (45.1, 5.1)
  line L26 (38.1, 3.3) -> (45.1, 3.3)
  line L27 (36.1, 3.2845) -> (36.1, 3.3)
  line L28 (48.1, -3.2) -> (30.6, -3.2) projected
  line L29 (48.1, 9.7) -> (48.1, -3.2)
  line L30 (44.1, 9.7) -> (48.1, 9.7)
  line L31 (44.1, 10.3) -> (44.1, 9.7)
  line L32 (12.6, 5.2) -> (28.6, 5.2)
  line L33 (28.6, 5.2) -> (28.6, 3.3)
  line L34 (28.6, 3.3) -> (14.6, 3.3)
  line L35 (12.6, 5.3) -> (12.6, 5.2)
  line L36 (29.5691, 3.3) -> (28.6, 3.3)
  line L37 (28.6, 3.3) -> (28.6, 5.2)
  line L38 (28.6, 5.2) -> (29.5691, 5.2)
  line L39 (29.5691, 5.2) -> (29.5691, 3.3)
  line L40 (12.6, 5.3) -> (14.6, 3.3)
  line L41 (43.1, -7.2086) -> (28.6368, -7.2086) projected
  line L42 (48.1, -3.2) -> (43.1, -3.2)
  line L43 (43.1, -3.2) -> (43.1, -7.2086)
  line L44 (43.1, -7.2086) -> (48.1, -7.2086)
  line L45 (48.1, -7.2086) -> (48.1, -3.2)
  line L46 (29.5691, 3.3) -> (28.6, 3.3)
  line L47 (27.2497, -3.2) -> (27.2497, -4.2) projected
  line L48 (43.1, -3.2) -> (43.1, -28.2) projected
  line L49 (38.1, 3.3) -> (38.1, -3.2)
  line L50 (38.1, 3.3) -> (31.6, -3.2)
  line L51 (-12.9, -3.2) -> (38.85, -3.2) projected
  line L52 (38.1, 3.3) -> (47.2924, 3.3) construction
  line L53 (31.6, -3.2) -> (38.1, -3.2)
  point P0 (40.6417, 4.3064)
  point P1 (12.6, 3.3)
  point P2 (12.6, 5.3)
  point P3 (43.1, -3.2)
  point P4 (28.6368, -3.2)
  point P5 (12.7, 5.2)
  point P6 (28.6, 3.7845)
  point P7 (31.6, -3.2)
  dimension "d106" = 16
  dimension "d108" = 2
  dimension "d109" = 2
  dimension "d140" = 2.6
  dimension "d141" = 0.6
  dimension "d142" = 0.4
  dimension "d143" = 1.2
  dimension "d144" = 2.6
  dimension "d145" = 0.4
  dimension "d146" = 1.8
  dimension "d148" = 6.5
  dimension "d150" = 6.5
  dimension "d151" = 135
  dimension "d152" = 4.5
  dimension "d153" = 0.4
  dimension "d154" = 0.4
  constraints: 85 end point, 7 parallel, 5 point on line, 4 horizontal, 4 perpendicular, 1 collinear, 1 equal length, 1 vertical
  measures "d106" distance of L33.end point (12.6, 3.3)
  measures "d108" distance of L35.start point (12.6, 3.3)
  measures "d109" distance of L34.end point (12.6, 3.3)
  measures "d140" distance between parallel lines of L30 L17
  measures "d141" distance of L30.start L16.end
  measures "d142" distance between parallel lines of L10 L30
  measures "d143" distance between parallel lines of L15 L10
  measures "d144" distance between parallel lines of L12 L15
  measures "d145" distance between parallel lines of L24 L12
  measures "d146" distance between parallel lines of L26 L24
  measures "d148" distance between parallel lines of L3 L34
  measures "d150" distance between parallel lines of L28 L26
  measures "d151" angle of L50 L52
  measures "d152" distance between parallel lines of L32 L20
  measures "d153" distance from line of L9.start L20
  measures "d154" distance between parallel lines of L24 L8
extrude "Extrusion19" add sketch "Skizze21" against normal up to surface (15 mm away) contours L43 L28 L45 L44 | L3 L49 L26 L25 L24 L23 L22 L39 L38 L32 L40 L21 L20 L19 L18 L17 L16 L31 L30 L29 L28 | L50 L49 L3 | L36 L33 L38 L39 | L34 L40 L32 L33 | L32 L21 L40
sketch "Skizze22" plane through (-37.7131, -1.3218, -40.6417) normal (-1, 0, 0) x (0, 0, 1)
  circle A0 centre (23.6, -7) radius 1.6 projected
  arc A1 (43.1, -4.95) -> (41.35, -3.2) centre (40.1, -6.2) ccw projected
  line L0 (43.1, -4.95) -> (43.1, -7.2086) projected
  line L1 (43.1, -7.2086) -> (48.1, -7.2086) projected
  line L2 (-12.9, -3.2) -> (31.6, -3.2) projected
  line L3 (-12.9, -8.95) -> (-12.9, -3.2) projected
  arc A2 (-12.9, -11.45) -> (-12.9, -8.95) centre (-9.9, -10.2) ccw projected
  line L4 (-12.9, -23.95) -> (-12.9, -11.45) projected
  arc A3 (-8.65, -28.2) -> (-12.9, -23.95) centre (-9.9, -25.2) ccw projected
  line L5 (-8.65, -28.2) -> (6.1749, -28.2) projected
  arc A4 (8.6749, -28.2) -> (6.1749, -28.2) centre (7.4249, -25.2) ccw projected
  line L6 (8.6749, -28.2) -> (38.85, -28.2) projected
  arc A5 (43.1, -23.95) -> (38.85, -28.2) centre (40.1, -25.2) ccw projected
  line L7 (43.1, -7.45) -> (43.1, -23.95) projected
  arc A6 (38.85, -3.2) -> (43.1, -7.45) centre (40.1, -6.2) ccw projected
  circle A7 centre (16.0766, 6.8) radius 1.4
  circle A8 centre (28.0766, 6.8) radius 1.4
  line L8 (12.6, 5.2) -> (12.7, 5.2) projected
  line L9 (12.7, 5.2) -> (14.6, 3.3) projected
  line L10 (48.1, -7.2086) -> (48.1, 9.7) projected
  line L11 (48.1, 9.7) -> (44.1, 9.7) projected
  line L12 (44.1, 9.7) -> (44.1, 10.3) projected
  line L13 (44.1, 10.3) -> (42.1, 12.3) projected
  line L14 (42.1, 12.3) -> (38.1, 12.3) projected
  line L15 (38.1, 12.3) -> (36.1, 10.3) projected
  line L16 (36.1, 10.3) -> (36.1, 9.7) projected
  line L17 (36.1, 9.7) -> (12.6, 9.7) projected
  line L18 (12.6, 9.7) -> (12.6, 5.2) projected
  line L19 (14.6, 3.3) -> (35.1, 3.3) projected
  line L20 (35.1, 3.3) -> (35.1, 5.1) projected
  line L21 (35.1, 5.1) -> (45.1, 5.1) projected
  line L22 (45.1, 5.1) -> (45.1, 3.3) projected
  line L23 (45.1, 3.3) -> (38.1, 3.3) projected
  line L24 (38.1, 3.3) -> (31.6, -3.2) projected
  line L25 (38.85, -3.2) -> (41.35, -3.2) projected
  point P0 (40.6417, 1.3218)
  dimension "d112" = 2.8
  dimension "d113" = 2.8
  dimension "d116" = 0
  dimension "d117" = 12
  constraints: 2 centre point, 2 coincident
  measures "d112" diameter of A7
  measures "d113" diameter of A8
  measures "d116" vertical distance of A7.centre A8.centre
  measures "d117" distance of A7.centre A8.centre
hole "Bohrung2" at (-37.7131, 5.4782, -24.5652) at (-37.7131, 5.4782, -12.5652) direction (1, 0, 0) diameter 2.8 end through all
sketch "Skizze23" plane through (-37.7131, 8.3782, -4.5417) normal (0, 1, 0) x (1, 0, 0)
  line L0 (15, 0) -> (15, 23.5) projected
  line L1 (0, 23.5) -> (15, 23.5) projected
  line L2 (0, 0) -> (0, 23.5) projected
  line L3 (0, 0) -> (15, 0) projected
  line L4 (15, 7.4632) -> (5, 7.4632) projected
  circle A0 centre (10.8873, 4.7935) radius 3
  point P0 (37.7131, -4.5417)
  dimension "d126" = 6
  constraints: 1 centre point
  measures "d126" diameter of A0
ref_plane "Arbeitsebene6" through (-37.7131, -0.5218, -10.0417) normal (0, -1, 0) x (1, 0, 0)
extrude "Extrusion20" cut sketch "Skizze23" against normal up to surface (8.9 mm away) contours A0 L4 | L4 A0
sketch "Skizze25" plane through (-22.7131, -17.0486, -6.0424) normal (1, 0, 0) x (0, 0, -1)
  circle A0 centre (10.9993, 8.7268) radius 1.6 projected
  line L0 (13.9993, 18.2768) -> (11.1993, 18.2768)
  line L1 (11.1993, 18.2768) -> (11.1993, 19.7768)
  line L2 (11.1993, 19.7768) -> (13.9993, 19.7768)
  line L3 (13.9993, 19.7768) -> (13.9993, 18.2768)
  line L4 (19.9993, 19.0268) -> (5.9993, 19.0268) projected
  line L5 (13.9993, 18.2768) -> (11.1993, 19.7768) construction
  line L6 (11.1993, 18.2768) -> (13.9993, 19.7768) construction
  line L7 (15.8493, 19.7768) -> (9.3493, 19.7768)
  line L8 (9.3493, 19.7768) -> (9.3493, 21.7768)
  line L9 (9.3493, 21.7768) -> (15.8493, 21.7768)
  line L10 (15.8493, 21.7768) -> (15.8493, 19.7768)
  line L11 (15.8493, 19.7768) -> (9.3493, 21.7768) construction
  line L12 (9.3493, 19.7768) -> (15.8493, 21.7768) construction
  point P0 (-6.0424, 17.0486)
  point P1 (12.5993, 19.0268)
  point P2 (5.9993, 18.5113)
  point P3 (12.5993, 20.7768)
  point P4 (12.5993, 19.7768)
  point P5 (5.9993, 19.0268)
  dimension "d134" = 1.5
  dimension "d135" = 6.5
  dimension "d136" = 2
  dimension "d139" = 0
  constraints: 24 end point, 6 midpoint, 4 parallel, 2 horizontal, 2 perpendicular, 2 other
  measures "d134" distance of L0.end L1.end
  measures "d135" distance of L8.end L9.end
  measures "d136" distance of L7.end L8.end
  measures "d139" horizontal distance of point (12.599, 19.027) point (12.599, 20.777)
extrude "Extrusion21" cut sketch "Skizze25" against normal through all contours L0 L1 L4 L3 | L4 L1 L2 L3 | L2 L7 L8 L9 L10
sketch "Skizze26" plane through (-37.7131, -1.3218, -40.6417) normal (-1, 0, 0) x (0, 0, 1)
  line L0 (23.4, 4.05) -> (23.4, 3.3) projected
  line L1 (23.4, 3.3) -> (35.1, 3.3) projected
  line L2 (35.1, 3.3) -> (35.1, 5.1) projected
  line L3 (35.1, 5.1) -> (45.1, 5.1) projected
  line L4 (45.1, 5.1) -> (45.1, 3.3) projected
  line L5 (45.1, 3.3) -> (38.1, 3.3) projected
  line L6 (38.1, 3.3) -> (31.6, -3.2) projected
  line L7 (-12.9, -3.2) -> (31.6, -3.2) projected
  line L8 (-12.9, -8.95) -> (-12.9, -3.2) projected
  arc A0 (-12.9, -11.45) -> (-12.9, -8.95) centre (-9.9, -10.2) ccw projected
  line L9 (-12.9, -23.95) -> (-12.9, -11.45) projected
  arc A1 (-8.65, -28.2) -> (-12.9, -23.95) centre (-9.9, -25.2) ccw projected
  line L10 (-8.65, -28.2) -> (6.1749, -28.2) projected
  arc A2 (8.6749, -28.2) -> (6.1749, -28.2) centre (7.4249, -25.2) ccw projected
  line L11 (8.6749, -28.2) -> (38.85, -28.2) projected
  arc A3 (43.1, -23.95) -> (38.85, -28.2) centre (40.1, -25.2) ccw projected
  line L12 (43.1, -7.45) -> (43.1, -23.95) projected
  arc A4 (38.85, -3.2) -> (43.1, -7.45) centre (40.1, -6.2) ccw projected
  line L13 (38.85, -3.2) -> (41.35, -3.2) projected
  arc A5 (43.1, -4.95) -> (41.35, -3.2) centre (40.1, -6.2) ccw projected
  line L14 (43.1, -4.95) -> (43.1, -7.2086) projected
  line L15 (43.1, -7.2086) -> (48.1, -7.2086) projected
  line L16 (48.1, -7.2086) -> (48.1, 9.7) projected
  line L17 (48.1, 9.7) -> (44.1, 9.7) projected
  line L18 (44.1, 9.7) -> (44.1, 10.3) projected
  line L19 (44.1, 10.3) -> (42.1, 12.3) projected
  line L20 (42.1, 12.3) -> (38.1, 12.3) projected
  line L21 (38.1, 12.3) -> (36.1, 10.3) projected
  line L22 (36.1, 10.3) -> (36.1, 9.7) projected
  line L23 (36.1, 9.7) -> (12.6, 9.7) projected
  line L24 (12.6, 9.7) -> (12.6, 5.2) projected
  line L25 (12.6, 5.2) -> (12.7, 5.2) projected
  line L26 (12.7, 5.2) -> (14.6, 3.3) projected
  line L27 (14.6, 3.3) -> (20.6, 3.3) projected
  line L28 (20.6, 3.3) -> (20.6, 4.05) projected
  line L29 (20.6, 4.05) -> (18.75, 4.05) projected
  line L30 (18.75, 4.05) -> (18.75, 6.05) projected
  line L31 (18.75, 6.05) -> (25.25, 6.05) projected
  line L32 (25.25, 6.05) -> (25.25, 4.05) projected
  line L33 (25.25, 4.05) -> (23.4, 4.05) projected
  circle A6 centre (16.0766, 6.8) radius 1.4 projected
  circle A7 centre (28.0766, 6.8) radius 1.4 projected
  circle A8 centre (23.6, -7) radius 1.6 projected
  line L34 (36.1, 6.1) -> (36.1, 5.5) projected
  line L35 (36.1, 5.5) -> (35.1, 5.5) projected
  line L36 (35.1, 5.5) -> (35.1, 9.3) projected
  line L37 (35.1, 9.3) -> (45.1, 9.3) projected
  line L38 (45.1, 9.3) -> (45.1, 5.5) projected
  line L39 (45.1, 5.5) -> (44.1, 5.5) projected
  line L40 (44.1, 5.5) -> (44.1, 6.1) projected
  line L41 (44.1, 6.1) -> (42.1, 8.1) projected
  line L42 (42.1, 8.1) -> (38.1, 8.1) projected
  line L43 (38.1, 8.1) -> (36.1, 6.1) projected
  circle A9 centre (16.0766, -7) radius 1.4
  arc A10 (19.9503, -4.2) -> (27.2497, -4.2) centre (23.6, -7) ccw projected
  circle A11 centre (28.2, -7) radius 1.4
  point P0 (40.6417, 1.3218)
  dimension "d155" = 2.8
  dimension "d156" = 2.8
  constraints: 2 centre point, 1 point on circle
  measures "d155" diameter of A9
  measures "d156" diameter of A11
extrude "Extrusion22" cut sketch "Skizze26" against normal blind 10 contours A11 A10 | A10 A11
sketch "Skizze27" plane through (-36.7131, -4.5218, -49.5417) normal (0, 1, 0) x (1, 0, 0)
  circle A0 centre (9.8873, -40.2065) radius 3 projected
  circle A1 centre (9.8873, -40.2065) radius 2.7175
  point P0 (36.7131, -49.5417)
  constraints: 1 centre point, 1 coincident
extrude "Extrusion23" add sketch "Skizze27" along normal blind 2 contours A1
equation "\"d59\" = d58"
equation "\"d60\" = d58"
equation "\"d61\" = d58"
equation "\"d64\" = d58"
equation "\"d65\" = d58"
